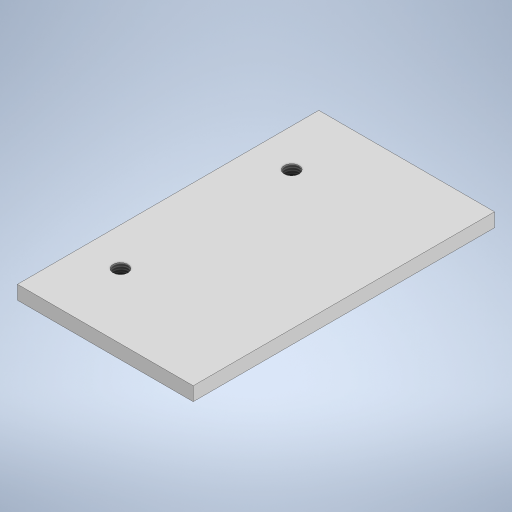
# Autodesk Inventor part: HL
Saved by Autodesk Inventor 2023 (Build 270158000, 158)
## iProperties
Created: 2022-10-24
Part Number: HL
Material: Generic
Document SubType Name: Modeling
Designer: User
Density: 1 g/cm^3
Appearance: Default
Author: User
Autodesk Inventor part; units mm, degrees
ref_plane "YZ Plane" through (0, 0, 0) normal (1, 0, 0) x (0, 1, 0)
ref_plane "XZ Plane" through (0, 0, 0) normal (0, 1, 0) x (-1, 0, 0)
ref_plane "XY Plane" through (0, 0, 0) normal (0, 0, 1) x (1, 0, 0)
sketch "Sketch1" plane through (0, 0, 0) normal (0, 1, 0) x (-1, 0, 0)
  line L0 (0, 0) -> (0, -120)
  line L1 (0, -120) -> (70, -120)
  line L2 (70, -120) -> (70, 0)
  line L3 (70, 0) -> (0, 0)
  line L4 (70, 0) -> (0, 0)
  dimension "d0" = 120
  dimension "d1" = 70
  constraints: 10 end point, 2 perpendicular, 1 collinear, 1 horizontal, 1 vertical
  measures "d0" distance of L0.start L0.end
  measures "d1" distance of L0.end L1.end
extrude "Extrusion1" add sketch "Sketch1" along normal blind 5.5
sketch "Sketch2" plane through (0, 5.5, 0) normal (0, 1, 0) x (1, 0, 0)
  line L0 (0, 120) -> (-70, 120) construction
  line L1 (0, 0) -> (0, 120) construction
  line L2 (-70, 120) -> (0, 0) construction
  line L3 (-70, 0) -> (0, 0) construction
  line L4 (-70, 0) -> (0, 120) construction
  line L5 (-70, 120) -> (-54.8839, 94.0866) construction
  line L6 (-70, 0) -> (-54.8839, 25.9134) construction
  dimension "d4" = 30
  dimension "d5" = 30
  constraints: 8 end point, 2 coincident, 2 point on line
  measures "d4" distance of L0.end L5.end
  measures "d5" distance of L3.start L6.end
hole "Hole1" at (-54.8839, 5.5, -94.0866) at (-54.8839, 5.5, -25.9134) direction (0, -1, 0) diameter 5.9175 depth 19.1 tip angle 118 thread size "M7x1" class "6H" standard "ANSI Metric M Profile"
body "Solid1"
